test_1 (Autodesk Fusion 360 design; units mm, degrees)
Autodesk Fusion 360 part; units mm, degrees
note: some values were not read from the file. Chosen so that the rebuilt part matches the saved one: which bodies a step acts on.
sketch "Sketch1" plane through (0, 0, 0) normal (0, 1, 0) x (1, 0, 0)
  line L0 (0, 0) -> (-20, 0)
  line L1 (-20, 0) -> (-20, -60)
  line L2 (-20, -60) -> (0, -60)
  line L3 (0, -60) -> (0, 0)
  line L4 (-5.5127, 0) -> (-13.6167, -8.6882)
  line L5 (-13.6167, -8.6882) -> (-8.0387, -18.2485)
  line L6 (-8.0387, -18.2485) -> (-19, -30)
  line L7 (-1, 0) -> (-9.5297, -9.1447)
  line L8 (-9.5297, -9.1447) -> (-3.9517, -18.7049)
  line L9 (-3.9517, -18.7049) -> (-14.4873, -30)
  line L10 (-13.6167, -8.6882) -> (-18.5619, -13.9899)
  arc A0 (-18.5619, -13.9899) -> (-9.3331, -16.0299) centre (-14.3, -16.6045) ccw
  line L11 (-9.5297, -9.1447) -> (-15.47, -15.5132)
  circle A1 centre (-14.3, -16.6045) radius 1.6
  line L12 (-11.8802, -11.6645) -> (-12.7205, -16.86)
  arc A2 (-10.9722, -26.2315) -> (-1.6266, -22.69) centre (-6.3603, -24.3) ccw
  line L13 (-8.0387, -18.2485) -> (-4.9784, -23.4937)
  line L14 (-3.9517, -18.7049) -> (-1.6266, -22.69)
  line L15 (-6.3022, -21.2248) -> (-7.7108, -23.442)
  circle A3 centre (-6.3603, -24.3) radius 1.6
  line L16 (0, -30) -> (-20, -30)
  line L17 (-10, -60) -> (-10, 0)
  dimension "d1" = 20
  dimension "d2" = 60
  dimension "d10" = 3.3
  dimension "d11" = 3.3
  dimension "d12" = 3.3
  dimension "d13" = 1
  dimension "d19" = 5
  dimension "d20" = 7.25
  dimension "d22" = 3.2
  dimension "d23" = 5.7
  dimension "d24" = 5.7
  dimension "d28" = 3.2
  dimension "d29" = 5
  dimension "d33" = 8.5
  dimension "d34" = 1
  dimension "d35" = 5.7
  constraint horizontal L0
  constraint vertical L1
  constraint horizontal L2
  constraint coincident L0.start L3.end
  constraint coincident L0 L4.start
  constraint parallel L4 L6
  constraint coincident L0 L7.start
  constraint parallel L5 L8
  constraint parallel L7 L9
  constraint parallel L6 L9
  constraint parallel L4 L10
  constraint coincident L10.end A0.start
  constraint coincident L5 A0.end
  constraint parallel L7 L11
  constraint concentric A0 A1
  constraint coincident L11.end A1
  constraint tangent L11 A1
  constraint coincident L5 L12.start
  constraint coincident L11 L12.start
  constraint coincident A1 L12.end
  constraint tangent A1 L12
  constraint collinear L8 L14
  constraint collinear L5 L13
  constraint coincident A2.end L14.end
  constraint coincident L9 A2.start
  constraint coincident L9 L15.start
  constraint coincident L15.start L13
  constraint tangent L15 A3
  constraint tangent L13 A3
  constraint coincident L13.end A3
  constraint coincident L15.end A3
  constraint concentric A2 A3
  constraint coincident L8.end L9.start
  constraint coincident L5.end L6.start
  constraint coincident L3 L16.start
  constraint coincident L1 L16.end
  constraint perpendicular L1 L16
  constraint midpoint L3 L16.start
  constraint perpendicular L0 L3
  constraint coincident L6.end L16
  constraint coincident L9.end L16
  constraint midpoint L2 L17.start
  constraint midpoint L0 L17.end
  measures "d1" distance of L0.start L0.end
  measures "d2" distance of L0.start L2.end
  measures "d10" distance of L6 L9
  measures "d11" distance of L5 L8
  measures "d12" distance of L4 L7
  measures "d13" distance of L0.start L7.start
  measures "d19" radius of A0
  measures "d20" distance of L4.end L10.end
  measures "d22" diameter of A1
  measures "d23" distance of L1 A0.centre
  measures "d24" distance of L6 A0.centre
  measures "d28" diameter of A3
  measures "d29" radius of A2
  measures "d33" distance of L4.end A0.end
  measures "d34" distance of L1 L6.end
  measures "d35" distance of A2.centre L16
extrude "Extrude1" add sketch "Sketch1" against normal blind 7 contours L0 L3 L7 L8 A2 L14 L16 L17 | L0 L4 L17 | L9 A2 L16 L17 | L0 L1 L4 L6 L10 A0 L16 L17 | L13 L15 A3 | L11 A1 L12 | L5 L6 A0 L17 | A3 | A1 makes body 1 at (-20, -2.3333, 10) makes body 2 at (-15.8977, -4.6667, 16.5182) makes body 3 at (0, -2.3333, 20) makes body 4 at (-7.9496, -4.6667, 24.4846)
pattern_linear "R-Pattern1" count 2 spacing 30 along (0, 0, 1) of bodies 3 1 2 4 makes body 5 at (-20, -2.3333, 50) makes body 6 at (-15.8016, -4.6667, 46.0521) makes body 7 at (0, -2.3333, 40) makes body 8 at (-7.9242, -2.3333, 54.6382)
ref_plane "WorkPlane1" through (-10, 0, 0) normal (1, 0, 0) x (0, 1, 0)
mirror "Mirror1" about plane through (-10, 0, 0) normal (1, 0, 0) of bodies 7 6 5 8 makes body 9 at (0, -2.3333, 50) makes body 10 at (-4.1984, -4.6667, 46.0521) makes body 11 at (-20, -2.3333, 40) makes body 12 at (-12.0941, -4.6667, 54.7139)
hidden bodies 5 6 7 8
equation "d9 = 3.3 mm"
equation "d10 = d9"
equation "d11 = d9"
equation "d12 = d9"
equation "d24 = d23"
equation "d28 = d22"
equation "d29 = d19"
equation "d35 = d23"
